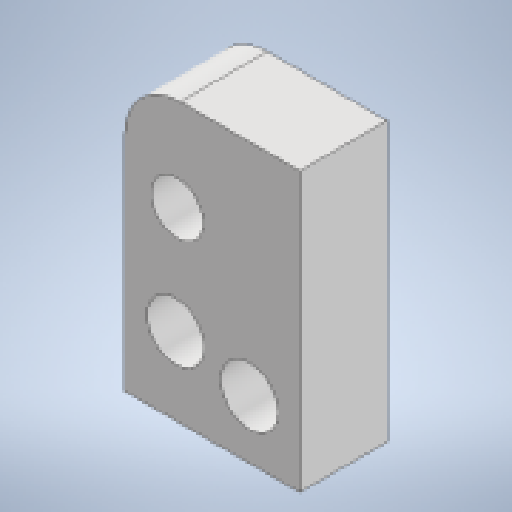
# Autodesk Inventor part: gates_top_holder
Saved by Autodesk Inventor 2025.2 (Build 292293000, 293)
## iProperties
Created: 2025-01-20
Part Number: gates_top_holder
Material: Типовые
Document SubType Name: Modeling
Designer: Admin
Density: 1 g/cm^3
Appearance: По умолчанию
Author: Admin
Autodesk Inventor part; units mm, degrees
ref_plane "YZ Plane" through (0, 0, 0) normal (1, 0, 0) x (0, 1, 0)
ref_plane "XZ Plane" through (0, 0, 0) normal (0, 1, 0) x (-1, 0, 0)
ref_plane "XY Plane" through (0, 0, 0) normal (0, 0, 1) x (1, 0, 0)
sketch "Эскиз1" plane through (0, 0, 0) normal (0, 0, 1) x (1, 0, 0)
  circle A0 centre (-2.1207, -4.0482) radius 1.65
  circle A1 centre (2.1207, -5.1509) radius 1.65
  line L0 (-5.0242, 4.325) -> (-5.0242, -8.5)
  line L1 (5.0242, -8.5) -> (5.0242, 7.5)
  line L2 (5.0242, 7.5) -> (-1.8492, 7.5)
  circle A2 centre (-2.0244, 2.1263) radius 1.5
  arc A3 (-1.8492, 7.5) -> (-5.0242, 4.325) centre (-1.8492, 4.325) ccw
  line L3 (-5.0242, -8.5) -> (5.0242, -8.5)
  dimension "d0" = 3.175
  dimension "d1" = 3.3
  dimension "d2" = 3
  dimension "d3" = 3.3
  constraints: 8 end point, 4 centre point, 2 point on circle, 2 tangent, 1 horizontal
  measures "d0" radius of A3
  measures "d1" diameter of A0
  measures "d2" diameter of A2
  measures "d3" diameter of A1
extrude "Выдавливание1" add sketch "Эскиз1" along normal blind 5
